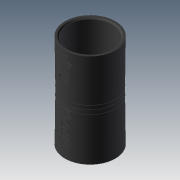
# Autodesk Inventor part: ExpToPeep
Saved by Autodesk Inventor 2020 (Build 240168000, 168)
## iProperties
Created: 2020-04-13
Part Number: ExpToPeep
Material: Generic
Document SubType Name: Modeling
Designer: Theo Cominotto
Density: 1 g/cm^3
Appearance: Default
Author: Theo Cominotto
Autodesk Inventor part; units mm, degrees
ref_plane "YZ Plane" through (0, 0, 0) normal (1, 0, 0) x (0, 1, 0)
ref_plane "XZ Plane" through (0, 0, 0) normal (0, 1, 0) x (-1, 0, 0)
sketch "Sketch2" plane through (0, 0, 0) normal (0, 0, 1) x (1, 0, 0)
  line L0 (0, 47) -> (-11.25, 47) construction
  line L1 (0, 47) -> (0, 22) construction
  line L2 (0, 22) -> (-10.5, 22) construction
  line L3 (-11.25, 47) -> (-11.035, 25.5)
  line L4 (-11.035, 25.5) -> (0, 25.5) construction
  line L5 (-11, 23.5) -> (11, 23.5) construction
  line L6 (-11.035, 25.5) -> (-11, 23.5)
  line L7 (-12.35, 23.5) -> (12.35, 23.5) construction
  line L8 (-11, 23.5) -> (-12.35, 23.5)
  line L9 (-12.35, 23.5) -> (-12.385, 25.5)
  line L10 (-12.385, 25.5) -> (-12.6, 47)
  line L11 (-12.6, 47) -> (-11.25, 47)
  line L12 (-11.035, 21.5) -> (0, 21.5) construction
  line L13 (-11.035, 21.5) -> (-11, 23.5)
  line L14 (-12.35, 23.5) -> (-12.385, 21.5)
  line L15 (0, 0) -> (0, 25) construction
  line L16 (0, 0) -> (-11.25, 0) construction
  line L17 (-11.25, 0) -> (-11.035, 21.5)
  line L18 (-12.385, 21.5) -> (-12.6, 0)
  line L19 (-12.6, 0) -> (-11.25, 0)
  line L20 (-17.59, 0) -> (17.34, 0) construction
  line L21 (0, -9.4) -> (0, 56.4) construction
  dimension "d0" = 11.25
  dimension "d1" = 25
  dimension "d2" = 10.5
  dimension "d3" = 3.5
  dimension "d4" = 2
  dimension "d5" = 90.573
  dimension "d6" = 1.35
  dimension "d14" = 179.57
  dimension "d15" = 179.57
  dimension "d16" = 179.57
  constraints: 40 end point, 7 symmetric about line, 4 point on line, 3 collinear, 3 horizontal, 1 parallel, 1 perpendicular
  measures "d0" distance of L1.start L0.end
  measures "d1" distance of L1.start L2.start
  measures "d2" distance of L2.start L2.end
  measures "d3" distance between parallel lines of L2 L4
  measures "d4" distance between parallel lines of L5 L4
  measures "d5" angle of L4 L3
  measures "d6" distance of L4.start L9.end
  measures "d14" angle of L6 L3
  measures "d15" angle of L10 L9
  measures "d16" angle of L18 L14
revolve "Revolution1" add sketch "Sketch2" angle 360 about axis through (0, 0, 0) along (0, 1, 0)
ref_plane "Work Plane1" through (0, 0, 12.75) normal (0, 0, 1) x (1, 0, 0)
sketch "Sketch3" plane through (0, 0, 12.75) normal (0, 0, 1) x (1, 0, 0)
  line L0 (-3.0784, 32.2065) -> (-3.0784, 43.2681) construction
  line L1 (-3.0784, 43.2681) -> (3.3033, 43.2681) construction
  line L2 (3.3033, 43.2681) -> (3.3033, 32.2065) construction
  line L3 (3.3033, 32.2065) -> (-3.0784, 32.2065) construction
  line L4 (12.385, 25.5) -> (-12.385, 25.5) projected
  line L5 (2.8546, 22.014) -> (2.8546, 10.9524) construction
  line L6 (2.8546, 10.9524) -> (-3.5271, 10.9524) construction
  line L7 (-3.5271, 10.9524) -> (-3.5271, 22.014) construction
  line L8 (-3.5271, 22.014) -> (2.8546, 22.014) construction
  line L9 (1.9216, 32.7251) -> (-3.0784, 32.7251)
  line L10 (-3.0784, 32.7251) -> (-3.0784, 36.1044)
  line L11 (-3.0784, 36.1044) -> (-2.1262, 36.1044)
  line L12 (-2.1262, 36.1044) -> (-2.1262, 33.9731)
  line L13 (-2.1262, 33.9731) -> (-1.247, 33.9731)
  line L14 (-1.247, 33.9731) -> (-1.247, 35.9382)
  line L15 (-1.247, 35.9382) -> (-0.2948, 35.9382)
  line L16 (-0.2948, 35.9382) -> (-0.2948, 33.9731)
  line L17 (-0.2948, 33.9731) -> (0.9694, 33.9731)
  line L18 (0.9694, 33.9731) -> (0.9694, 36.1044)
  line L19 (0.9694, 36.1044) -> (1.9216, 36.1044)
  line L20 (1.9216, 36.1044) -> (1.9216, 32.7251)
  line L21 (1.9216, 40.606) -> (1.9216, 39.2284)
  line L22 (1.9216, 39.2284) -> (0.8397, 38.5112)
  line L23 (0.8397, 38.5112) -> (1.9216, 37.7737)
  line L24 (1.9216, 37.7737) -> (1.9216, 36.4245)
  line L25 (1.9216, 36.4245) -> (0.0334, 37.8143)
  line L26 (0.0334, 37.8143) -> (-1.8507, 36.4488)
  line L27 (-1.8507, 36.4488) -> (-1.8507, 37.8264)
  line L28 (-1.8507, 37.8264) -> (-0.7891, 38.5314)
  line L29 (-0.7891, 38.5314) -> (-1.8507, 39.2405)
  line L30 (-1.8507, 39.2405) -> (-1.8507, 40.5898)
  line L31 (-1.8507, 40.5898) -> (0.0051, 39.2243)
  line L32 (0.0051, 39.2243) -> (1.9216, 40.606)
  spline S0 degree 2 poles (-0.0152, 44.7389) (0.8884, 44.7389) (1.9945, 43.8232) (1.9945, 43.1506) knots 0 0 0 1 2 2 2
  spline S1 degree 2 poles (1.9945, 43.1506) (1.9945, 42.871) (1.8689, 42.4536) (1.7312, 42.2186) knots 0 0 0 1 2 2 2
  line L33 (1.7312, 42.2186) -> (3.3033, 42.2186)
  line L34 (3.3033, 42.2186) -> (3.3033, 41.0436)
  line L35 (3.3033, 41.0436) -> (-1.8507, 41.0436)
  line L36 (-1.8507, 41.0436) -> (-1.8507, 42.2186)
  line L37 (-1.8507, 42.2186) -> (-1.4536, 42.2186)
  spline S2 degree 2 poles (-1.4536, 42.2186) (-1.6765, 42.478) (-1.952, 43.0128) (-1.952, 43.3653) knots 0 0 0 1 2 2 2
  spline S3 degree 2 poles (-1.952, 43.3653) (-1.952, 44.0217) (-0.9107, 44.7389) (-0.0152, 44.7389) knots 0 0 0 1 2 2 2
  spline S4 degree 2 poles (0.0091, 43.5355) (-0.5419, 43.5355) (-1.0363, 43.1951) (-1.0363, 42.8386) knots 0 0 0 1 2 2 2
  spline S5 degree 2 poles (-1.0363, 42.8386) (-1.0363, 42.6805) (-0.935, 42.3686) (-0.8337, 42.2186) knots 0 0 0 1 2 2 2
  line L38 (-0.8337, 42.2186) -> (1.0585, 42.2186)
  spline S6 degree 2 poles (1.0585, 42.2186) (1.0991, 42.3118) (1.1315, 42.5387) (1.1315, 42.6927) knots 0 0 0 1 2 2 2
  spline S7 degree 2 poles (1.1315, 42.6927) (1.1315, 43.1181) (0.5723, 43.5355) (0.0091, 43.5355) knots 0 0 0 1 2 2 2
  spline S8 degree 2 poles (1.2784, 17.6501) (0.93, 17.6501) (0.2979, 17.873) (0.0872, 18.0796) knots 0 0 0 1 2 2 2
  spline S9 degree 2 poles (0.0872, 18.0796) (-0.0465, 18.2052) (-0.2653, 18.5132) (-0.3423, 18.6955) knots 0 0 0 1 2 2 2
  spline S10 degree 2 poles (-0.3423, 18.6955) (-0.4193, 18.8819) (-0.5084, 19.3154) (-0.5084, 19.5829) knots 0 0 0 1 2 2 2
  line L39 (-0.5084, 19.5829) -> (-0.5084, 20.2393)
  line L40 (-0.5084, 20.2393) -> (-2.1454, 20.2393)
  line L41 (-2.1454, 20.2393) -> (-2.1454, 21.4954)
  line L42 (-2.1454, 21.4954) -> (2.8546, 21.4954)
  line L43 (2.8546, 21.4954) -> (2.8546, 19.5545)
  spline S11 degree 2 poles (2.8546, 19.5545) (2.8546, 19.125) (2.6966, 18.497) (2.5264, 18.2417) knots 0 0 0 1 2 2 2
  spline S12 degree 2 poles (2.5264, 18.2417) (2.336, 17.9581) (1.712, 17.6501) (1.2784, 17.6501) knots 0 0 0 1 2 2 2
  spline S13 degree 2 poles (1.246, 18.9386) (1.4608, 18.9386) (1.7647, 19.1412) (1.8214, 19.279) knots 0 0 0 1 2 2 2
  spline S14 degree 2 poles (1.8214, 19.279) (1.8984, 19.4573) (1.9227, 19.7814) (1.9227, 20.061) knots 0 0 0 1 2 2 2
  line L44 (1.9227, 20.061) -> (1.9227, 20.2393)
  line L45 (1.9227, 20.2393) -> (0.4235, 20.2393)
  line L46 (0.4235, 20.2393) -> (0.4235, 20.1501)
  spline S15 degree 2 poles (0.4235, 20.1501) (0.4235, 19.9759) (0.4316, 19.6599) (0.4519, 19.5424) knots 0 0 0 1 2 2 2
  spline S16 degree 2 poles (0.4519, 19.5424) (0.4681, 19.4411) (0.5653, 19.2182) (0.6261, 19.1574) knots 0 0 0 1 2 2 2
  spline S17 degree 2 poles (0.6261, 19.1574) (0.7477, 19.0278) (1.0191, 18.9386) (1.246, 18.9386) knots 0 0 0 1 2 2 2
  spline S18 degree 2 poles (-2.2467, 15.1137) (-2.2467, 16.1834) (-1.2256, 17.3219) (-0.2815, 17.3219) knots 0 0 0 1 2 2 2
  spline S19 degree 2 poles (-0.2815, 17.3219) (0.6423, 17.3219) (1.7444, 16.2603) (1.7444, 15.3041) knots 0 0 0 1 2 2 2
  spline S20 degree 2 poles (1.7444, 15.3041) (1.7444, 14.4411) (0.8084, 13.5659) (-0.0587, 13.5659) knots 0 0 0 1 2 2 2
  line L47 (-0.0587, 13.5659) -> (-0.4841, 13.5659)
  line L48 (-0.4841, 13.5659) -> (-0.4841, 16.1469)
  spline S21 degree 2 poles (-0.4841, 16.1469) (-0.7475, 16.1307) (-1.0959, 15.9402) (-1.2013, 15.7863) knots 0 0 0 1 2 2 2
  spline S22 degree 2 poles (-1.2013, 15.7863) (-1.3066, 15.6364) (-1.3958, 15.2312) (-1.3958, 14.9921) knots 0 0 0 1 2 2 2
  spline S23 degree 2 poles (-1.3958, 14.9921) (-1.3958, 14.7895) (-1.3066, 14.3924) (-1.2297, 14.2263) knots 0 0 0 1 2 2 2
  spline S24 degree 2 poles (-1.2297, 14.2263) (-1.1689, 14.0804) (-1.019, 13.8373) (-0.9622, 13.7603) knots 0 0 0 1 2 2 2
  line L49 (-0.9622, 13.7603) -> (-0.9622, 13.6347)
  line L50 (-0.9622, 13.6347) -> (-1.9347, 13.6347)
  spline S25 degree 2 poles (-1.9347, 13.6347) (-1.9914, 13.7806) (-2.0887, 14.0156) (-2.1373, 14.2263) knots 0 0 0 1 2 2 2
  spline S26 degree 2 poles (-2.1373, 14.2263) (-2.19, 14.4167) (-2.2467, 14.8219) (-2.2467, 15.1137) knots 0 0 0 1 2 2 2
  spline S27 degree 2 poles (0.225, 14.7247) (0.5977, 14.7328) (0.9908, 15.061) (0.9908, 15.3973) knots 0 0 0 1 2 2 2
  spline S28 degree 2 poles (0.9908, 15.3973) (0.9908, 15.7417) (0.5775, 16.1307) (0.225, 16.1509) knots 0 0 0 1 2 2 2
  line L51 (0.225, 16.1509) -> (0.225, 14.7247)
  spline S29 degree 2 poles (-2.2467, 11.0294) (-2.2467, 12.0991) (-1.2256, 13.2377) (-0.2815, 13.2377) knots 0 0 0 1 2 2 2
  spline S30 degree 2 poles (-0.2815, 13.2377) (0.6423, 13.2377) (1.7444, 12.1761) (1.7444, 11.2198) knots 0 0 0 1 2 2 2
  spline S31 degree 2 poles (1.7444, 11.2198) (1.7444, 10.3568) (0.8084, 9.4816) (-0.0587, 9.4816) knots 0 0 0 1 2 2 2
  line L52 (-0.0587, 9.4816) -> (-0.4841, 9.4816)
  line L53 (-0.4841, 9.4816) -> (-0.4841, 12.0626)
  spline S32 degree 2 poles (-0.4841, 12.0626) (-0.7475, 12.0464) (-1.0959, 11.856) (-1.2013, 11.702) knots 0 0 0 1 2 2 2
  spline S33 degree 2 poles (-1.2013, 11.702) (-1.3066, 11.5521) (-1.3958, 11.1469) (-1.3958, 10.9078) knots 0 0 0 1 2 2 2
  spline S34 degree 2 poles (-1.3958, 10.9078) (-1.3958, 10.7052) (-1.3066, 10.3082) (-1.2297, 10.142) knots 0 0 0 1 2 2 2
  spline S35 degree 2 poles (-1.2297, 10.142) (-1.1689, 9.9962) (-1.019, 9.753) (-0.9622, 9.6761) knots 0 0 0 1 2 2 2
  line L54 (-0.9622, 9.6761) -> (-0.9622, 9.5505)
  line L55 (-0.9622, 9.5505) -> (-1.9347, 9.5505)
  spline S36 degree 2 poles (-1.9347, 9.5505) (-1.9914, 9.6963) (-2.0887, 9.9313) (-2.1373, 10.142) knots 0 0 0 1 2 2 2
  spline S37 degree 2 poles (-2.1373, 10.142) (-2.19, 10.3325) (-2.2467, 10.7377) (-2.2467, 11.0294) knots 0 0 0 1 2 2 2
  spline S38 degree 2 poles (0.225, 10.6404) (0.5977, 10.6485) (0.9908, 10.9767) (0.9908, 11.313) knots 0 0 0 1 2 2 2
  spline S39 degree 2 poles (0.9908, 11.313) (0.9908, 11.6574) (0.5775, 12.0464) (0.225, 12.0667) knots 0 0 0 1 2 2 2
  line L56 (0.225, 12.0667) -> (0.225, 10.6404)
  spline S40 degree 2 poles (-0.2086, 5.1825) (-1.1122, 5.1825) (-2.2183, 6.0983) (-2.2183, 6.7709) knots 0 0 0 1 2 2 2
  spline S41 degree 2 poles (-2.2183, 6.7709) (-2.2183, 7.0505) (-2.0927, 7.4678) (-1.9549, 7.7028) knots 0 0 0 1 2 2 2
  line L57 (-1.9549, 7.7028) -> (-3.5271, 7.7028)
  line L58 (-3.5271, 7.7028) -> (-3.5271, 8.8778)
  line L59 (-3.5271, 8.8778) -> (1.6269, 8.8778)
  line L60 (1.6269, 8.8778) -> (1.6269, 7.7028)
  line L61 (1.6269, 7.7028) -> (1.2298, 7.7028)
  spline S42 degree 2 poles (1.2298, 7.7028) (1.4527, 7.4435) (1.7282, 6.9086) (1.7282, 6.5561) knots 0 0 0 1 2 2 2
  spline S43 degree 2 poles (1.7282, 6.5561) (1.7282, 5.8997) (0.6869, 5.1825) (-0.2086, 5.1825) knots 0 0 0 1 2 2 2
  spline S44 degree 2 poles (-0.2329, 6.3859) (0.3182, 6.3859) (0.8125, 6.7263) (0.8125, 7.0829) knots 0 0 0 1 2 2 2
  spline S45 degree 2 poles (0.8125, 7.0829) (0.8125, 7.2409) (0.7112, 7.5529) (0.6099, 7.7028) knots 0 0 0 1 2 2 2
  line L62 (0.6099, 7.7028) -> (-1.2823, 7.7028)
  spline S46 degree 2 poles (-1.2823, 7.7028) (-1.3229, 7.6096) (-1.3553, 7.3827) (-1.3553, 7.2287) knots 0 0 0 1 2 2 2
  spline S47 degree 2 poles (-1.3553, 7.2287) (-1.3553, 6.8033) (-0.7961, 6.3859) (-0.2329, 6.3859) knots 0 0 0 1 2 2 2
  point P0 (0, 0)
  constraints: 2 parallel, 4 other
extrude "Extrusion1" add sketch "Sketch3" against normal up to surface
sketch "Sketch4" plane through (0, 0, 0) normal (1, 0, 0) x (0, 1, 0)
  line L0 (47, 11.25) -> (25.5, 11.035) projected
  line L1 (47, -11.25) -> (47, 11.25) projected
  line L2 (47, 11.1) -> (25.5, 10.885)
  line L3 (25.5, -11.035) -> (25.5, 11.035) projected
  line L4 (-9.4, 0) -> (56.4, 0) projected
  point P0 (0, 0)
  dimension "d17" = 0.15
  constraints: 2 end point, 2 point on line, 1 parallel
  measures "d17" distance of L0.end L2.end
revolve "Revolution2" add sketch "Sketch4" angle 360 about axis through (0, -10, 0) along (0, 1, 0) contours L1 L2 L3 L0
chamfer "Chamfer2" distance 0.6 angle 45 2 edges at (11.25, 0, 0) (0, 47, -11.1)
chamfer "Chamfer3" distance 0.15 angle 45 1 edges at (0, 25.5, -10.885)
equation "\"d4\" = d7"
equation "\"d6\" = d8"
equation "\"d7\" = 2"
equation "\"d8\" = 1.35"
equation "\"d9\" = 0"
body "Solid1"
